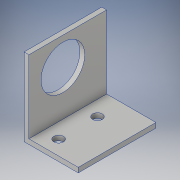
# Autodesk Inventor part: CLB_090_ClimberMotorBearingBracket
Saved by Autodesk Inventor 2018 (Build 220112000, 112)
## iProperties
Created: 2020-03-01
Part Number: CLB_090_ClimberMotorBearingBracket
Material: Aluminum 6061
Document SubType Name: Modeling
Designer: Cooper
Density: 2.7 g/cm^3
Appearance: Aluminum - Flat
Author: Cooper
Autodesk Inventor part; units mm, degrees
ref_plane "YZ Plane" through (0, 0, 0) normal (1, 0, 0) x (0, 1, 0)
ref_plane "XZ Plane" through (0, 0, 0) normal (0, 1, 0) x (-1, 0, 0)
ref_plane "XY Plane" through (0, 0, 0) normal (0, 0, 1) x (1, 0, 0)
sketch "Sketch1" plane through (0, 0, 0) normal (0, 0, 1) x (1, 0, 0)
  line L0 (0, 0) -> (0, 50.8)
  line L1 (0, 50.8) -> (3.175, 50.8)
  line L2 (3.175, 50.8) -> (3.175, 3.175)
  line L3 (3.175, 3.175) -> (35.433, 3.175)
  line L4 (35.433, 3.175) -> (35.433, 0)
  line L5 (35.433, 0) -> (0, 0)
  dimension "d0" = 50.8
  dimension "d1" = 35.433
  dimension "d2" = 3.175
  dimension "d3" = 3.175
  constraints: 12 end point, 5 perpendicular, 1 vertical
  measures "d0" distance of L0.start L0.end
  measures "d1" distance of L4.end L0.start
  measures "d2" distance between parallel lines of L2 L0
  measures "d3" distance of L3.end L4.end
extrude "Extrusion1" add sketch "Sketch1" along normal blind 47.625 and the other way blind 3.2004
sketch "Sketch2" plane through (0, 0, -3.2004) normal (-1, 0, 0) x (0, 0, 1)
  line L0 (0, 0) -> (0, 50.8) projected
  line L1 (0, 0) -> (50.8254, 0) projected
  line L2 (50.8254, 50.8) -> (50.8254, 0) projected
  line L3 (50.8254, 50.8) -> (0, 50.8) projected
  point P0 (3.2004, 0)
  point P1 (28.6004, 32.5438)
  dimension "d6" = 28.6004
  dimension "d8" = 32.5438
  measures "d6" distance from line of L0 point (28.6, 32.544)
  measures "d8" distance from line of L1 point (28.6, 32.544)
hole "Hole1" at (0, 32.5438, 25.4) direction (1, 0, 0) diameter 28.575 end through all
sketch "Sketch4" plane through (0, 0, 47.625) normal (0, -1, 0) x (1, 0, 0)
  line L0 (35.433, -50.8254) -> (0, -50.8254) projected
  line L1 (35.433, 0) -> (35.433, -50.8254) projected
  point P0 (0, -47.625)
  point P1 (13.0556, -34.9504)
  point P2 (13.0556, -9.5504)
  dimension "d29" = 15.875
  dimension "d30" = 22.3774
  dimension "d31" = 25.4
  dimension "d32" = 22.3774
  measures "d29" distance from line of point (13.056, -34.95) L0
  measures "d30" distance from line of point (13.056, -34.95) L1
  measures "d31" distance of point (13.056, -9.55) point (13.056, -34.95)
  measures "d32" distance from line of L1 point (13.056, -9.55)
hole "Hole3" at (13.0556, 0, 12.6746) at (13.0556, 0, 38.0746) direction (0, 1, 0) diameter 6.35 end through all
equation "\"d3\" = d2"
body "Solid1"
